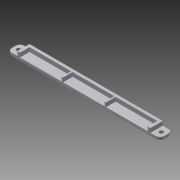
# Autodesk Inventor part: base_corner
Saved by Autodesk Inventor 2014 SP1 (Build 180222100, 222)
## iProperties
Created: 2016-08-31
Part Number: base_corner
Material: ABS Plastic
Document SubType Name: Modeling
Designer: tguillod
Density: 1.06 g/cm^3
Appearance: Smooth - White
Author: tguillod
Autodesk Inventor part; units mm, degrees
ref_plane "YZ Plane" through (0, 0, 0) normal (1, 0, 0) x (0, 1, 0)
ref_plane "XZ Plane" through (0, 0, 0) normal (0, 1, 0) x (-1, 0, 0)
ref_plane "XY Plane" through (0, 0, 0) normal (0, 0, 1) x (1, 0, 0)
sketch "Sketch1" plane through (0, 0, 0) normal (0, 0, 1) x (1, 0, 0)
  line L0 (0, 0) -> (97.5, 0)
  line L1 (97.5, 0) -> (97.5, 9)
  line L2 (97.5, 9) -> (0, 9)
  line L3 (0, 9) -> (0, 0)
  dimension "d2" = 97.5
  dimension "d3" = 9
  constraints: 8 end point, 2 parallel, 1 horizontal, 1 perpendicular
  measures "d2" distance of L1.end L2.end
  measures "d3" distance of L0.end L1.end
extrude "Extrusion1" add sketch "Sketch1" along normal blind 5
sketch "Sketch2" plane through (0, 0, 5) normal (0, 0, 1) x (1, 0, 0)
  line L0 (0, 0) -> (97.5, 0) projected
  line L1 (97.5, 0) -> (97.5, 9) projected
  line L2 (0, 9) -> (0, 0) projected
  line L3 (2, 0) -> (32.5, 0)
  line L4 (32.5, 0) -> (32.5, 7)
  line L5 (32.5, 7) -> (2, 7)
  line L6 (2, 7) -> (2, 0)
  line L7 (33.5, 7) -> (64, 7)
  line L8 (64, 7) -> (64, 0)
  line L9 (64, 0) -> (33.5, 0)
  line L10 (33.5, 0) -> (33.5, 7)
  line L11 (65, 0) -> (95.5, 0)
  line L12 (95.5, 0) -> (95.5, 7)
  line L13 (95.5, 7) -> (65, 7)
  line L14 (65, 7) -> (65, 0)
  dimension "d4" = 7
  dimension "d5" = 30.5
  dimension "d6" = 2
  dimension "d7" = 2
  dimension "d8" = 30.5
  dimension "d9" = 30.5
  dimension "d10" = 1
  constraints: 24 end point, 6 parallel, 3 horizontal, 3 perpendicular, 3 point on line, 2 collinear
  measures "d4" distance of L5.end L3.start
  measures "d5" distance of L4.end L5.end
  measures "d6" distance between parallel lines of L6 L2
  measures "d7" distance between parallel lines of L1 L12
  measures "d8" distance of L12.end L13.end
  measures "d9" distance of L7.start L7.end
  measures "d10" distance between parallel lines of L10 L4
extrude "Extrusion2" cut sketch "Sketch2" against normal blind 3
sketch "Sketch3" plane through (0, 0, 0) normal (-1, 0, 0) x (0, 0, 1)
  line L0 (0, 9) -> (0, 0) projected
  line L1 (0, 0) -> (5, 0) projected
  line L2 (0, 9) -> (2, 9)
  line L3 (2, 9) -> (2, 0)
  line L4 (2, 0) -> (0, 0)
  line L5 (0, 0) -> (0, 9)
  dimension "d13" = 2
  constraints: 8 end point, 2 parallel, 1 horizontal, 1 perpendicular, 1 point on line
  measures "d13" distance of L0.start L2.end
extrude "Extrusion3" add sketch "Sketch3" along normal blind 7
sketch "Sketch5" plane through (97.5, 0, 0) normal (1, 0, 0) x (0, 0, -1)
  line L0 (0, 0) -> (-5, 0) projected
  line L1 (0, 9) -> (-2, 9)
  line L2 (-2, 9) -> (-2, 0)
  line L3 (-2, 0) -> (0, 0)
  line L4 (0, 0) -> (0, 9)
  dimension "d22" = 2
  constraints: 8 end point, 2 parallel, 1 horizontal, 1 perpendicular, 1 point on line
  measures "d22" distance of L1.start L1.end
extrude "Extrusion5" add sketch "Sketch5" along normal blind 7
sketch "Sketch7" plane through (0, 0, 2) normal (0, 0, 1) x (1, 0, 0)
  line L0 (-7, 0) -> (-7, 9) projected
  line L1 (97.5, 0) -> (97.5, 9) projected
  line L2 (97.5, 0) -> (104.5, 0) projected
  line L3 (104.5, 9) -> (104.5, 0) projected
  line L4 (97.5, 9) -> (104.5, 9) projected
  point P0 (-3.5, 4.5)
  point P1 (101, 4.5)
  dimension "d31" = 3.5
  dimension "d32" = 4.5
  dimension "d33" = 3.5
  measures "d31" distance from line of L0 point (-3.5, 4.5)
  measures "d32" distance from line of point (101, 4.5) L4
  measures "d33" distance from line of L3 point (101, 4.5)
hole "Hole1" at (-3.5, 4.5, 2) at (101, 4.5, 2) direction (0, 0, -1) diameter 3 end through all
fillet "Fillet1" radius 3 4 edges at (104.5, 0, 1) (104.5, 9, 1) (-7, 0, 1) (-7, 9, 1)
body "Solid1"
